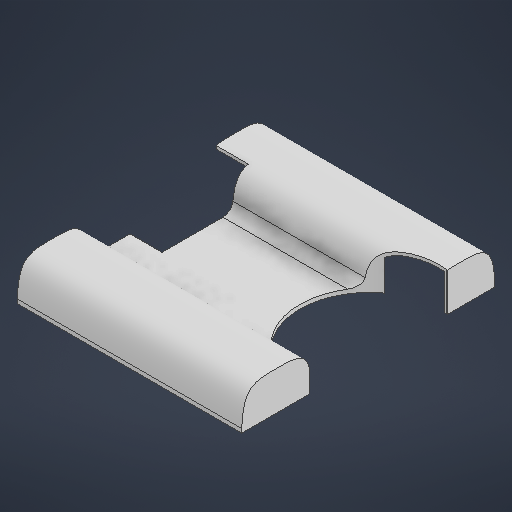
# Autodesk Inventor part: DebrisCover
Saved by Autodesk Inventor 2026.2 (Build 302298000, 298)
## iProperties
Created: 2026-02-16
Part Number: DebrisCover
Material: Generic
Document SubType Name: Modeling
Designer: Thomas
Density: 1 g/cm^3
Appearance: Default
Author: Thomas
Autodesk Inventor part; units mm, degrees
ref_plane "YZ Plane" through (0, 0, 0) normal (1, 0, 0) x (0, 1, 0)
ref_plane "XZ Plane" through (0, 0, 0) normal (0, 1, 0) x (-1, 0, 0)
ref_plane "XY Plane" through (0, 0, 0) normal (0, 0, 1) x (1, 0, 0)
sketch "Sketch1" plane through (0, 0, 0) normal (1, 0, 0) x (0, 1, 0)
  line L0 (-2.54, 84.1375) -> (2.54, 84.1375)
  line L1 (2.54, 84.1375) -> (2.54, -84.1375)
  line L2 (2.54, -84.1375) -> (-2.54, -84.1375)
  line L3 (-2.54, -84.1375) -> (-2.54, 84.1375)
  line L4 (-2.54, 84.1375) -> (2.54, -84.1375) construction
  line L5 (2.54, 84.1375) -> (-2.54, -84.1375) construction
  spline S0 degree 4 poles (2.54, 71.4375) (86.5501, 75.2143) (7.7052, 115.8875) (86.5501, 156.5607) (2.54, 160.3375) knots 0 0 0 0 0 1 1 1 1 1
  line L6 (2.54, 160.3375) -> (-2.54, 160.3375)
  line L7 (-2.54, 160.3375) -> (-2.54, 147.6375)
  line L8 (-2.54, 147.6375) -> (2.54, 147.6375)
  line L9 (2.54, 147.6375) -> (2.54, 160.3375)
  line L10 (2.54, 147.6375) -> (36.5375, 147.6375)
  line L11 (2.54, 84.1375) -> (36.5375, 84.1375)
  spline S1 degree 4 poles (2.54, -160.3375) (86.9132, -156.5846) (7.2211, -115.8875) (86.9132, -75.1904) (2.54, -71.4375) knots 0 0 0 0 0 1 1 1 1 1
  line L12 (2.54, -84.1375) -> (36.6323, -84.1375)
  line L13 (2.54, -147.6375) -> (36.6323, -147.6375)
  line L14 (2.54, -160.3375) -> (-2.54, -160.3375)
  line L15 (-2.54, -160.3375) -> (-2.54, -147.6375)
  line L16 (-2.54, -147.6375) -> (2.54, -147.6375)
  line L17 (2.54, -147.6375) -> (2.54, -160.3375)
  spline S2 degree 5 poles (2.3689, 75.2437) (2.4031, 75.2452) (2.4373, 75.2468) (2.4716, 75.2483) (2.5058, 75.2499) (2.54, 75.2514) knots 0 0 0 0 0 0 1 1 1 1 1 1
  spline S3 degree 5 poles (36.5375, 84.1376) (37.0443, 84.6384) (37.5226, 85.168) (37.9688, 85.7258) (39.2068, 87.4829) (40.1328, 89.4325) (40.6164, 90.7887) (41.4529, 93.7789) (41.9283, 96.8506) (42.116, 98.5088) (42.4097, 102.0198) (42.5484, 105.5394) (42.5965, 107.3923) (42.6608, 111.1606) (42.6762, 114.9297) (42.6762, 116.8453) (42.6608, 120.6144) (42.5965, 124.3827) (42.5484, 126.2356) (42.4097, 129.7552) (42.116, 133.2662) (41.9283, 134.9244) (41.4529, 137.9961) (40.6164, 140.9863) (40.1328, 142.3425) (39.2068, 144.2921) (37.9688, 146.0492) (37.5226, 146.607) (37.0443, 147.1366) (36.5375, 147.6374) knots 0 0 0 0 0 0 0.053781 0.053781 0.053781 0.1619 0.1619 0.1619 0.287839 0.287839 0.287839 0.427709 0.427709 0.427709 0.572291 0.572291 0.572291 0.712161 0.712161 0.712161 0.8381 0.8381 0.8381 0.946219 0.946219 0.946219 1 1 1 1 1 1
  spline S4 degree 5 poles (2.54, 156.5236) (2.5058, 156.5251) (2.4716, 156.5267) (2.4373, 156.5282) (2.4031, 156.5298) (2.3689, 156.5313) knots 0 0 0 0 0 0 1 1 1 1 1 1
  spline S5 degree 5 poles (36.6322, -147.6374) (37.1338, -147.1396) (37.6068, -146.6132) (38.0479, -146.0589) (39.2766, -144.3055) (40.1926, -142.3603) (40.6704, -141.0046) (41.4955, -138.0134) (41.96, -134.942) (42.1425, -133.2827) (42.4265, -129.7686) (42.5577, -126.2463) (42.6026, -124.3915) (42.662, -120.6193) (42.6758, -116.8463) (42.6758, -114.9287) (42.662, -111.1557) (42.6026, -107.3835) (42.5577, -105.5287) (42.4265, -102.0064) (42.1425, -98.4923) (41.96, -96.833) (41.4955, -93.7616) (40.6704, -90.7704) (40.1926, -89.4147) (39.2766, -87.4695) (38.0479, -85.7161) (37.6068, -85.1618) (37.1338, -84.6354) (36.6322, -84.1376) knots 0 0 0 0 0 0 0.053378 0.053378 0.053378 0.161389 0.161389 0.161389 0.287464 0.287464 0.287464 0.427576 0.427576 0.427576 0.572424 0.572424 0.572424 0.712536 0.712536 0.712536 0.838611 0.838611 0.838611 0.946622 0.946622 0.946622 1 1 1 1 1 1
  point P0 (0, 0)
  point P1 (44.45, 90.4875)
  point P2 (46.482, 115.8875)
  point P3 (44.45, 141.2875)
  point P4 (44.5065, -141.2875)
  point P5 (46.482, -115.8875)
  point P6 (44.5065, -90.4875)
  point P7 (2.54, -71.4375)
  dimension "d0" = 5.08
  dimension "d1" = 168.275
  dimension "d2" = 12.7
  dimension "d3" = 88.9
  dimension "d4" = 44.45
  dimension "d5" = 43.942
  dimension "d6" = 19.05
  dimension "d7" = 19.05
  dimension "d8" = 5.08
  dimension "d9" = 12.7
  dimension "d13" = 12.7
  dimension "d14" = 88.9
  dimension "d15" = 44.45
  dimension "d16" = 43.942
  dimension "d17" = 19.05
  dimension "d18" = 19.05
  dimension "d21" = 63.5
  dimension "d22" = 5.08
  dimension "d23" = 12.7
  constraints: 36 end point, 8 vertical alignment, 7 horizontal, 6 parallel, 5 point on line, 3 perpendicular, 2 midpoint, 20 other
  measures "d0" distance of L1.end L2.end
  measures "d1" distance of L0.end L1.end
  measures "d2" distance of L0.end point (2.54, 71.438)
  measures "d3" distance of L6.start point (2.54, 71.438)
  measures "d4" vertical distance of point (46.482, 115.888) point (2.54, 71.438)
  measures "d5" horizontal distance of point (46.482, 115.888) L0.end
  measures "d6" vertical distance of point (44.45, 141.288) L6.start
  measures "d7" vertical distance of point (44.45, 90.487) point (2.54, 71.438)
  measures "d8" distance of L8.end L7.end
  measures "d9" distance of L7.end L6.end
  measures "d13" distance of L13.start L14.start
  measures "d14" distance of point (2.54, -71.438) L14.start
  measures "d15" vertical distance of point (46.482, -115.888) L14.start
  measures "d16" horizontal distance of point (46.482, -115.888) L13.start
  measures "d17" vertical distance of point (44.507, -90.487) point (2.54, -71.438)
  measures "d18" vertical distance of point (44.507, -141.288) L14.start
  measures "d21" distance between parallel lines of L13 L12
  measures "d22" distance of L15.end L16.end
  measures "d23" distance of L14.end L15.end
extrude "Extrusion1" add sketch "Sketch1" against normal blind 284.48
fillet "Fillet1" radius 12.7 2 edges at (-142.24, 2.54, 71.4375) (-142.24, 2.54, -71.4375)
sketch "Sketch5" plane through (0, 0, 0) normal (1, 0, 0) x (0, 0, -1)
  line L0 (-150.8125, -2.54) -> (-150.8125, 34.925)
  line L1 (-150.8125, 34.925) -> (-147.6375, 39.6875)
  line L2 (-147.6375, 39.6875) -> (-131.7625, 44.45)
  line L3 (-131.7625, 44.45) -> (-93.6625, 44.45)
  line L4 (-93.6625, 44.45) -> (-84.1375, 39.6875)
  line L5 (-84.1375, 39.6875) -> (-79.375, 28.575)
  line L6 (-79.375, 28.575) -> (-79.375, -2.54)
  line L7 (84.1375, -2.54) -> (-84.1375, -2.54) projected
  line L8 (80.9625, -2.54) -> (80.9625, 37.3062)
  line L9 (80.9625, 37.3062) -> (93.6625, 42.8625)
  line L10 (93.6625, 42.8625) -> (138.1125, 44.45)
  line L11 (138.1125, 44.45) -> (149.225, 37.3062)
  line L12 (149.225, 37.3062) -> (150.6481, -2.54)
  line L13 (80.9625, -2.54) -> (150.6481, -2.54)
  line L14 (160.3375, -2.54) -> (147.6375, -2.54) projected
  line L15 (-150.8125, -2.54) -> (-79.375, -2.54)
  point P0 (0, 0)
  constraints: 28 end point, 2 collinear, 2 perpendicular, 2 vertical, 1 horizontal, 1 point on line
extrude "Extrusion4" add sketch "Sketch5" against normal blind 3.81
sketch "Sketch6" plane through (0, 2.54, 59.6855) normal (0, 1, 0) x (1, 0, 0)
  line L0 (0, 59.6855) -> (0, 72.3855) construction
  line L1 (0, 119.3627) -> (0, 0) projected
  line L2 (39.6875, 160.0155) -> (-11.1125, -15.2445) construction
  line L3 (-10.2851, 157.1611) -> (39.6875, -15.2445) construction
  line L4 (39.6875, -15.2445) -> (39.6875, -12.1458)
  arc A0 (35.9343, -2.2959) -> (39.6875, 0.2047) centre (-11.1125, 72.3855) ccw
  arc A1 (-0.544, 160.0155) -> (-0.544, -15.2445) centre (-11.1125, 72.3855) ccw
  arc A2 (29.119, -15.2445) -> (29.119, 160.0155) centre (39.6875, 72.3855) ccw
  arc A3 (-7.3593, 147.0669) -> (-11.1125, 144.5663) centre (39.6875, 72.3855) ccw
  line L5 (-11.1125, 156.9169) -> (-11.1125, 144.5663)
  line L6 (-11.1125, -12.1458) -> (-11.1125, -15.2445)
  arc A4 (38.8601, -12.39) -> (39.6875, -12.1458) centre (14.2875, 72.3855) ccw
  arc A5 (24.856, 160.0155) -> (3.719, 160.0155) centre (14.2875, 72.3855) ccw
  arc A6 (-10.2851, 157.1611) -> (-11.1125, 156.9169) centre (14.2875, 72.3855) ccw
  arc A7 (-11.1125, -12.1458) -> (-10.2851, -12.39) centre (14.2875, 72.3855) ccw
  arc A8 (3.719, -15.2445) -> (24.856, -15.2445) centre (14.2875, 72.3855) ccw
  line L7 (29.119, 160.0155) -> (24.856, 160.0155)
  line L8 (3.719, 160.0155) -> (-11.1125, 160.0155)
  line L9 (-0.544, -15.2445) -> (3.719, -15.2445)
  line L10 (24.856, -15.2445) -> (29.119, -15.2445)
  dimension "d62" = 12.7
  dimension "d63" = 50.8
  dimension "d64" = 175.26
  constraints: 20 end point, 18 point on circle, 9 centre point, 7 point on line, 6 parallel, 4 perpendicular, 2 horizontal, 1 coincident, 1 horizontal alignment, 1 midpoint
  measures "d62" distance of L0.start L0.end
  measures "d63" distance of L3.end L2.end
  measures "d64" distance of L2.end L8.end
extrude "Extrusion9" cut sketch "Sketch6" along normal through all both and the other way through all
sketch "Sketch7" plane through (-284.48, 2.54, 59.6855) normal (0, 1, 0) x (1, 0, 0)
  line L0 (0, 42.223) -> (40.64, 42.223)
  line L1 (40.64, 42.223) -> (40.64, 151.443)
  line L2 (40.64, 151.443) -> (0, 151.443)
  line L3 (0, 151.443) -> (0, 42.223)
  line L4 (0, 42.223) -> (40.64, 151.443) construction
  line L5 (40.64, 42.223) -> (0, 151.443) construction
  line L6 (284.48, 220.023) -> (0, 220.023) projected
  line L7 (0, 0) -> (0, 119.3627) projected
  point P0 (284.48, 59.6855)
  point P1 (20.32, 96.833)
  point P2 (20.32, 151.443)
  dimension "d70" = 40.64
  dimension "d71" = 109.22
  dimension "d72" = 68.58
  dimension "d73" = 0
  constraints: 12 end point, 3 midpoint, 2 parallel, 1 horizontal, 1 perpendicular
  measures "d70" distance of L2.end L1.end
  measures "d71" distance of L1.end L0.end
  measures "d72" distance from line of point (20.32, 151.443) L6
  measures "d73" distance between parallel lines of L7 L3
extrude "Extrusion10" cut sketch "Sketch7" along normal through all both and the other way through all
body "Solid1"
